# Autodesk Inventor part: Zahnriemen
Saved by Autodesk Inventor 2016 (Build 200138000, 138)
## iProperties
Created: 2015-08-10
Part Number: Zahnriemen
Material: Rubber
Document SubType Name: Modeling
Designer: 4ndreas
Density: 1 g/cm^3
Appearance: Rubber - Black - Version 1.1
CustomPartVersion: 1
Author: 4ndreas
Autodesk Inventor part; units mm, degrees
sketch "Skizzenpfad" plane through (0, 0, 0) normal (0, 0, 1) x (1, 0, 0)
  arc A0 (41.3576, -50.4735) -> (-44.7764, -47.4668) centre (0, 0) ccw
  arc A1 (11.9309, -74.5855) -> (9.5443, -81.5633) centre (16.3675, -80) ccw
  arc A2 (-12.7203, -97.4733) -> (12.4108, -94.0745) centre (0, -96.918) ccw
  arc A3 (-13.4964, -79.6947) -> (-15.6864, -74.9081) centre (-20.4897, -80) ccw
  line L0 (-15.6864, -74.9081) -> (-44.7764, -47.4668)
  line L1 (41.3576, -50.4735) -> (11.9309, -74.5855)
  line L2 (9.5443, -81.5633) -> (12.4108, -94.0745)
  line L3 (-12.7203, -97.4733) -> (-13.4964, -79.6947)
  constraints: 8 end point, 6 point on circle, 3 centre point, 3 other
ref_plane "Querschnittsebene" through (-44.7764, -47.4668, 0) normal (0.7274, -0.6862, 0) x (0, 0, 1)
ref_plane "Arbeitsebene2" through (0, 0, 0) normal (-1, 0, 0) x (0, 0, 1)
ref_plane "Arbeitsebene3" through (0, -96.918, 0) normal (-0.1347, 0.9909, 0) x (0, 0, 1)
sketch "Querschnitt" plane through (-44.7764, -47.4668, 0) normal (0.7274, -0.6862, 0) x (0, 0, 1)
  line L0 (-5, 0.5) -> (5, 0.5)
  line L1 (5, 0.5) -> (5, -0.5)
  line L2 (5, -0.5) -> (-5, -0.5)
  line L3 (-5, -0.5) -> (-5, 0.5)
  line L4 (-5, 0) -> (5, 0) construction
  point P0 (0, 0)
  point P1 (0, 0)
  dimension "d0" = 10
  dimension "d4" = 0.5
  dimension "d5" = 0.5
  constraints: 10 end point, 3 midpoint, 2 parallel, 1 coincident, 1 horizontal, 1 perpendicular, 1 other
  measures "d0" distance between parallel lines of L1 L3
  measures "d4" distance between parallel lines of L2 L4
  measures "d5" distance between parallel lines of L4 L0
sweep "Riemen" add profiles "Querschnitt" path "Skizzenpfad"
equation "\"d0\" = da_B"
equation "\"d4\" = da_a"
equation "\"d5\" = da_a2"
equation "\"da_B\" = 10"
equation "\"da_pb\" = 5"
equation "\"da_a\" = 0.5"
equation "\"da_S\" = 2.65"
equation "\"da_Beta\" = 20deg"
equation "\"da_Ht\" = 1.2"
equation "\"da_H\" = 2.2"
equation "\"da_a2\" = 0.5"
body "Solid1"
